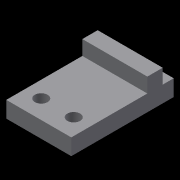
# Autodesk Inventor part: slider v1
Saved by Autodesk Inventor 2015 SP1 (Build 190203100, 203)
## iProperties
Created: 2014-12-05
Part Number: slider v1
Material: Generic
Document SubType Name: Modeling
Designer: datenney
Density: 1 g/cm^3
Appearance: Default
Author: datenney
Autodesk Inventor part; units mm, degrees
ref_plane "YZ Plane" through (0, 0, 0) normal (1, 0, 0) x (0, 1, 0)
ref_plane "XZ Plane" through (0, 0, 0) normal (0, 1, 0) x (-1, 0, 0)
ref_plane "XY Plane" through (0, 0, 0) normal (0, 0, 1) x (1, 0, 0)
sketch "Sketch1" plane through (0, 0, 0) normal (0, 1, 0) x (-1, 0, 0)
  line L0 (0, 0) -> (25.4, 0)
  line L1 (25.4, 0) -> (25.4, -40.005)
  line L2 (25.4, -40.005) -> (0, -40.005)
  line L3 (0, -40.005) -> (0, 0)
  dimension "d0" = 40.005
  dimension "d1" = 25.4
  constraints: 8 end point, 2 parallel, 1 horizontal, 1 perpendicular
  measures "d0" distance of L0.end L1.end
  measures "d1" distance between parallel lines of L3 L1
extrude "Extrusion1" add sketch "Sketch1" along normal blind 6.35
sketch "Sketch2" plane through (0, 6.35, 0) normal (0, 1, 0) x (1, 0, 0)
  line L0 (-25.4, 40.005) -> (-25.4, 0) projected
  line L1 (0, 0) -> (0, 40.005) projected
  line L2 (-25.4, 35.6997) -> (0, 35.6997)
  line L3 (0, 35.6997) -> (0, 29.7053)
  line L4 (0, 29.7053) -> (-25.4, 29.7053)
  line L5 (-25.4, 29.7053) -> (-25.4, 35.6997)
  line L6 (-25.4, 32.7025) -> (0, 32.7025) construction
  line L7 (-25.4, 7.3025) -> (0, 7.3025)
  line L8 (-25.4, 0) -> (0, 0) projected
  line L9 (0, 40.005) -> (-25.4, 40.005) projected
  line L10 (-25.4, 29.7053) -> (0, 29.7053)
  line L11 (0, 29.7053) -> (0, 35.6997)
  line L12 (0, 35.6997) -> (-25.4, 35.6997)
  line L13 (-25.4, 35.6997) -> (-25.4, 29.7053)
  point P0 (-19.05, 7.3025)
  point P1 (-6.35, 7.3025)
  dimension "d4" = 5.9944
  dimension "d5" = 25.4
  dimension "d6" = 7.3025
  dimension "d7" = 40.005
  dimension "d8" = 12.7
  dimension "d9" = 25.4
  dimension "d10" = 6.35
  constraints: 20 end point, 6 point on line, 4 parallel, 3 horizontal, 2 midpoint, 2 perpendicular
  measures "d4" distance between parallel lines of L4 L2
  measures "d5" distance between parallel lines of L6 L7
  measures "d6" distance between parallel lines of L8 L7
  measures "d7" distance between parallel lines of L8 L9
  measures "d8" distance of point (-19.05, 7.302) point (-6.35, 7.302)
  measures "d9" distance between parallel lines of L1 L0
  measures "d10" distance of L7.start point (-19.05, 7.302)
extrude "Extrusion2" add sketch "Sketch2" along normal blind 5.715 contours L2 L1 L4 L0
hole "Hole1" at (-19.05, 6.35, -7.3025) at (-6.35, 6.35, -7.3025) direction (0, -1, 0) diameter 5 end through all
equation "\"d6\" = -0.5 * d5 + 0.5 * d7"
equation "\"d10\" = -0.5 * d8 + 0.5 * d9"
body "Solid1"
